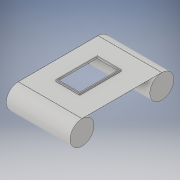
# Autodesk Inventor part: conveyar_belt
Saved by Autodesk Inventor 2019 (Build 230136000, 136)
## iProperties
Created: 2020-02-19
Part Number: conveyar_belt
Material: Generic
Document SubType Name: Sheet Metal
Designer: HP
Density: 1 g/cm^3
Sheet Metal Rule: Default_mm
Appearance: Default
Author: HP
Autodesk Inventor part; units mm, degrees
ref_plane "YZ Plane" through (0, 0, 0) normal (1, 0, 0) x (0, 1, 0)
ref_plane "XY Plane" through (0, 0, 0) normal (0, 0, 1) x (1, 0, 0)
sketch "Sketch1" plane through (0, 0, 0) normal (1, 0, 0) x (0, 1, 0)
  circle A0 centre (0, 0) radius 75
  circle A1 centre (0, -500) radius 75
  dimension "d0" = 150
  dimension "d1" = 150
  dimension "d2" = 500
  constraints: 2 centre point, 1 coincident
  measures "d0" diameter of A0
  measures "d1" diameter of A1
  measures "d2" distance of A1.centre point (0, 0)
extrude "Extrusion1" add sketch "Sketch1" along normal blind 400
ref_plane "Work Plane1" through (0, 75, -500) normal (0, 1, 0) x (-1, 0, 0)
sketch "Sketch2" plane through (0, 75, -500) normal (0, 1, 0) x (-1, 0, 0)
  line L0 (-400, 75) -> (-400, -75)
  line L1 (0, 500) -> (-400, 500)
  line L2 (-400, 500) -> (-400, 0)
  line L3 (-400, 0) -> (0, 0)
  line L4 (0, 0) -> (0, 500)
sheet face with bend "Face1" sketch "Sketch2" thickness 0.5 toward (0, 1, 0) bend radius 0.5 relief straight relief width 0.5 relief depth 0.25
bend "Bend1"
sketch "Sketch3" plane through (0, 75.5, -500) normal (0, 1, 0) x (1, 0, 0)
  line L0 (116.3614, -380.5646) -> (266.5244, -380.5646)
  line L1 (266.5244, -380.5646) -> (266.5244, -121.0916)
  line L2 (266.5244, -121.0916) -> (116.3614, -121.0916)
  line L3 (116.3614, -121.0916) -> (116.3614, -380.5646)
  point P0 (0, -500)
  constraints: 8 end point, 2 parallel, 1 horizontal, 1 perpendicular
extrude "Extrusion2" cut sketch "Sketch3" against normal blind 2
sketch "Sketch4" plane through (0, 75.5, -500) normal (0, 1, 0) x (1, 0, 0)
  line L0 (116.3614, -380.5646) -> (116.3614, -121.0916) projected
  line L1 (266.5244, -380.5646) -> (116.3614, -380.5646)
  line L2 (116.3614, -380.5646) -> (116.3614, -121.0916)
  line L3 (116.3614, -121.0916) -> (266.5244, -121.0916)
  line L4 (266.5244, -121.0916) -> (266.5244, -380.5646)
  point P0 (0, -500)
  constraints: 8 end point, 2 parallel, 1 horizontal, 1 perpendicular
extrude "Extrusion3" add sketch "Sketch4" along normal blind 10
sketch "Sketch5" plane through (0, 85.5, -500) normal (0, 1, 0) x (1, 0, 0)
  line L0 (260.3624, -374.3919) -> (120.8007, -374.3919)
  line L1 (120.8007, -374.3919) -> (120.8007, -126.4749)
  line L2 (120.8007, -126.4749) -> (260.3624, -126.4749)
  line L3 (260.3624, -126.4749) -> (260.3624, -374.3919)
  point P0 (0, -500)
  constraints: 8 end point, 2 parallel, 1 horizontal, 1 perpendicular
extrude "Extrusion4" cut sketch "Sketch5" against normal blind 10
equation "\"d5\" = Thickness"
equation "\"d6\" = BendRadius"
equation "\"d7\" = BendReliefWidth"
equation "\"d9\" = MinimumRemnant"
equation "\"d8\" = BendReliefDepth"
equation "\"d10\" = TransitionRadius"
equation "\"BendRadius\" = Thickness"
equation "\"BendReliefWidth\" = Thickness"
equation "\"BendReliefDepth\" = 0.5 * Thickness"
equation "\"CornerReliefSize\" = 4 * Thickness"
equation "\"MinimumRemnant\" = 2 * Thickness"
equation "\"TransitionRadius\" = BendRadius"
equation "\"JacobiRadiusSize\" = BendRadius"
equation "\"GapSize\" = Thickness"
equation "\"Thickness\" = 0.5"
body "Solid1"
